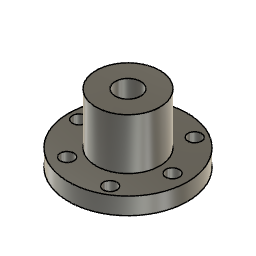
法兰联轴器 v3 (Autodesk Fusion 360 design; units mm, degrees)
Autodesk Fusion 360 part; units mm, degrees
note: some values were not read from the file. Set by a fixed rule: which sketch regions a step uses.
sketch "草图1" plane through (0, 0, 0) normal (0, 0, 1) x (1, 0, 0)
  circle A0 centre (0, 0) radius 14
  dimension "d1" = 28
  constraint coincident A0.centre origin
  measures "d1" diameter of A0
extrude "拉伸1" add sketch "草图1" along normal blind 4 makes body 1
sketch "草图2" plane through (0, 0, 4) normal (0, 0, 1) x (-1, 0, 0)
  circle A0 centre (0, 0) radius 14
  circle A1 centre (0, 0) radius 11.5 construction
  line L0 (13, 0) -> (-13, 0)
  circle A2 centre (11.5, 0) radius 1.6
  circle A3 centre (-5.75, 9.9593) radius 1.6
  circle A4 centre (-5.75, -9.9593) radius 1.6
  circle A5 centre (0, 0) radius 10.5 construction
  circle A6 centre (-10.5, 0) radius 1.6
  circle A7 centre (5.25, -9.0933) radius 1.6
  circle A8 centre (5.25, 9.0933) radius 1.6
  dimension "d4" = 23
  dimension "d5" = 3.2
  dimension "d7" = 360
  dimension "d8" = 21
  dimension "d9" = 3.2
  dimension "d11" = 360
  constraint coincident A0.centre A1.centre
  constraint horizontal L0
  constraint coincident A1 A2.centre
  constraint coincident L0 A2.centre
  constraint coincident A0.centre L0
  constraint coincident A5 A6.centre
  constraint coincident L0 A6.centre
  measures "d4" diameter of A1
  measures "d5" diameter of A2
  measures "d8" diameter of A5
  measures "d9" diameter of A6
extrude "拉伸2" cut sketch "草图2" against normal blind 4 contours L0 A6 | L0 A6 | A2 | A3 | A4 | A7 | A8 bodies 1
sketch "草图3" plane through (0, 0, 4) normal (0, 0, 1) x (-1, 0, 0)
  circle A0 centre (-5.75, -9.9593) radius 1.6
  circle A1 centre (11.5, 0) radius 1.6
  circle A2 centre (-10.5, 0) radius 1.6
  circle A3 centre (5.25, 9.0933) radius 1.6
  circle A4 centre (5.25, -9.0933) radius 1.6
  circle A5 centre (-5.75, 9.9593) radius 1.6
  circle A6 centre (0, 0) radius 14
  circle A7 centre (0, 0) radius 7.5
  dimension "d14" = 15
  constraint coincident A6.centre A7.centre
  measures "d14" diameter of A7
extrude "拉伸3" add sketch "草图3" along normal blind 12 contours A7 bodies 1
sketch "草图4" plane through (0, 0, 16) normal (0, 0, 1) x (-1, 0, 0)
  circle A0 centre (0, 0) radius 7.5
  circle A1 centre (0, 0) radius 3
  dimension "d17" = 6
  constraint coincident A0.centre A1.centre
  measures "d17" diameter of A1
extrude "拉伸4" cut sketch "草图4" against normal blind 16 contours A1 bodies 1
ref_plane "工作平面1" through (0, 8, 0) normal (0, 1, 0) x (0, 0, 1)
sketch "草图5" plane through (0, 8, 0) normal (0, 1, 0) x (1, 0, 0)
  line L0 (0, -14) -> (0, 7)
  circle A0 centre (0, -8) radius 2
  dimension "d21" = 4
  dimension "d22" = 8
  constraint vertical L0
  constraint coincident L0 A0.centre
  measures "d21" diameter of A0
  measures "d22" distance of origin A0.centre
extrude "拉伸5" cut sketch "草图5" against normal blind 8 bodies 1
copy_body "实体->零部件1" bodies 1 removing the originals makes body 2 in component "Component'"
component "Component'" placed x (1, 0, 0) y (0, 1, 0) z (0, 0, 1) at (0, 0, 0)
